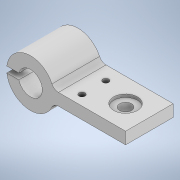
# Autodesk Inventor part: HingeGuide
Saved by Autodesk Inventor 2022.2 (Build 262287030, 287C)
## iProperties
Created: 2023-03-29
Part Number: HingeGuide
Material: Generic
Document SubType Name: Modeling
Designer: jak27277
Mass: 119.301 g
Surface Area: 261.005 cm^2
Volume: 119.301 cm^3
Density: 1 g/cm^3
Appearance: Default
Author: jak27277
Autodesk Inventor part; units mm, degrees
ref_plane "YZ Plane" through (0, 0, 0) normal (1, 0, 0) x (0, 1, 0)
ref_plane "XZ Plane" through (0, 0, 0) normal (0, 1, 0) x (-1, 0, 0)
ref_plane "XY Plane" through (0, 0, 0) normal (0, 0, 1) x (1, 0, 0)
sketch "Sketch1" plane through (0, 0, 0) normal (0, 0, 1) x (1, 0, 0)
  circle A0 centre (0, 0) radius 25.4
  line L0 (101.6, -6.35) -> (24.5934, -6.35)
  line L1 (24.5934, -6.35) -> (24.5934, 6.35) construction
  line L2 (24.5934, 6.35) -> (101.6, 6.35)
  line L3 (101.6, 6.35) -> (101.6, -6.35)
  line L4 (101.6, -6.35) -> (24.5934, 6.35) construction
  line L5 (24.5934, -6.35) -> (101.6, 6.35) construction
  circle A1 centre (0, 0) radius 12.7
  line L6 (-25.4, -3.175) -> (-12.2967, -3.175)
  line L7 (-12.2967, -3.175) -> (-12.2967, 3.175)
  line L8 (-12.2967, 3.175) -> (-25.4, 3.175)
  line L9 (-25.4, 3.175) -> (-25.4, -3.175)
  line L10 (-25.4, -3.175) -> (-12.2967, 3.175) construction
  line L11 (-12.2967, -3.175) -> (-25.4, 3.175) construction
  point P0 (63.0967, 0)
  point P1 (-18.8484, 0)
  point P2 (-25.2008, 3.175)
  point P3 (-25.2008, -3.175)
  dimension "d0" = 50.8
  dimension "d3" = 25.4
  dimension "d1" = 12.7
  dimension "d2" = 6.35
  dimension "d4" = 101.6
  constraints: 24 end point, 4 midpoint, 4 parallel, 2 coincident, 2 horizontal, 2 horizontal alignment, 2 perpendicular, 1 vertical, 6 other
  measures "d1" distance of L2.end L0.start
  measures "d2" distance of L8.end L6.start
  measures "d4" distance from line of point (0, 0) L3
extrude "Extrusion1" add sketch "Sketch1" along normal mid plane 50.8 contours A0 L6 A1 L8 | A0 L2 L3 L0 picked at (17.6529, 11.4324)
sketch "Sketch2" plane through (24.5934, 6.35, 25.4) normal (0, 1, 0) x (1, 0, 0)
  line L0 (77.0066, 50.8) -> (77.0066, 0) projected
  line L1 (0, 50.8) -> (77.0066, 50.8) projected
  point P0 (-24.5934, 25.4)
  point P1 (51.6066, 25.4)
  dimension "d7" = 25.4
  dimension "d8" = 25.4
  measures "d7" distance from line of L0 point (51.607, 25.4)
  measures "d8" distance from line of L1 point (51.607, 25.4)
hole "Hole1" at (76.2, 6.35, 0) direction (0, -1, 0) diameter 12.7 end through all counterbore diameter 25.4 counterbore depth 3.175
sketch "Sketch3" plane through (24.5934, 6.35, 25.4) normal (0, 1, 0) x (1, 0, 0)
  line L0 (77.0066, 50.8) -> (77.0066, 0) projected
  point P0 (-24.5934, 25.4)
  point P1 (19.8566, 10.6326)
  point P2 (19.8566, 36.0326)
  dimension "d16" = 25.4
  dimension "d17" = 57.15
  constraints: 1 vertical alignment
  measures "d16" distance of point (19.857, 10.633) point (19.857, 36.033)
  measures "d17" distance from line of L0 point (19.857, 10.633)
hole "Hole2" at (44.45, 6.35, 14.7674) at (44.45, 6.35, -10.6326) direction (0, -1, 0) diameter 6.35 end through all
fillet "Fillet1" radius 7.62 2 edges at (24.5934, 6.35, 0) (24.5934, -6.35, 0)
body "Solid1"
